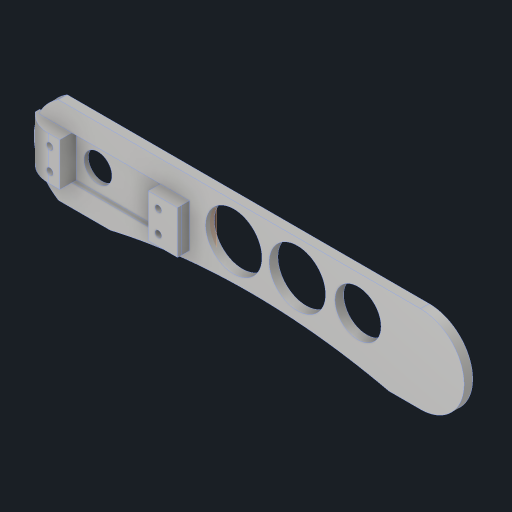
# Autodesk Inventor part: elbow
Saved by Autodesk Inventor 2023.4 (Build 274418000, 418)
## iProperties
Created: 2020-06-03
Part Number: elbow
Material: Aluminum 6061
Document SubType Name: Modeling
Designer: lenovo
Density: 2.7 g/cm^3
Appearance: Aluminum - Flat
Author: lenovo
Autodesk Inventor part; units mm, degrees
ref_plane "YZ Plane" through (0, 0, 0) normal (1, 0, 0) x (0, 1, 0)
ref_plane "XZ Plane" through (0, 0, 0) normal (0, 1, 0) x (-1, 0, 0)
ref_plane "XY Plane" through (0, 0, 0) normal (0, 0, 1) x (1, 0, 0)
sketch "Sketch1" plane through (0, 0, 0) normal (0, 0, 1) x (1, 0, 0)
  line L0 (-43.3376, 0) -> (106.6624, 0) construction
  line L1 (-43.3376, -20) -> (106.6624, -20)
  line L2 (106.6624, 20) -> (-43.3376, 20)
  arc A0 (-43.3376, 20) -> (-43.3376, -20) centre (-43.3376, 0) ccw
  arc A1 (106.6624, -20) -> (106.6624, 20) centre (106.6624, 0) ccw
  point P0 (0, 0)
  point P1 (31.6624, 0)
  dimension "d0" = 150
  dimension "d1" = 20
  constraints: 8 end point, 4 point on circle, 4 tangent, 2 centre point, 1 horizontal, 1 midpoint, 1 parallel
  measures "d0" distance of L0.end L0.start
  measures "d1" radius of A1
extrude "Extrusion1" add sketch "Sketch1" along normal blind 4
sketch "Sketch2" plane through (0, 0, 4) normal (0, 0, 1) x (1, 0, 0)
  arc A0 (-43.3376, 20) -> (-43.3376, -20) centre (-43.3376, 0) ccw projected
  arc A1 (106.6624, -20) -> (106.6624, 20) centre (106.6624, 0) ccw projected
  circle A2 centre (-43.3376, 0) radius 6.4
  circle A3 centre (106.6624, 0) radius 4
  point P0 (0, 0)
  dimension "d4" = 12.8
  dimension "d5" = 8
  constraints: 2 centre point, 2 coincident
  measures "d4" diameter of A2
  measures "d5" diameter of A3
extrude "Extrusion2" add sketch "Sketch2" against normal blind 11.9 contours A3
sketch "Sketch5" plane through (0, 0, 4) normal (0, 0, 1) x (1, 0, 0)
  line L0 (-43.3376, -20) -> (106.6624, -20) projected
  arc A0 (92.1536, -20) -> (-35.7554, -20) centre (28.1991, -294.1981) ccw
  point P0 (0, 0)
  constraints: 2 point on circle, 2 point on line, 1 centre point
extrude "Extrusion5" cut sketch "Sketch5" against normal through all
sketch "Sketch6" plane through (0, 0, 0) normal (0, 0, -1) x (-1, 0, 0)
  point P0 (0, 0)
sketch "Sketch7" plane through (106.6624, 0, -7.9) normal (0, 0, -1) x (-1, 0, 0)
  circle A0 centre (0, 0) radius 2.7
  point P0 (106.6624, 0)
  dimension "d18" = 5.4
  constraints: 1 centre point
  measures "d18" diameter of A0
extrude "Extrusion6" cut sketch "Sketch7" against normal blind 5
sketch "Sketch8" plane through (0, 0, 0) normal (0, 0, -1) x (-1, 0, 0)
  point P0 (0, 0)
extrude "Extrusion7" cut sketch "Sketch2" along normal mid plane 11.9 contours A2
sketch "Sketch9" plane through (106.6624, 0, -7.9) normal (0, 0, -1) x (-1, 0, 0)
  point P0 (106.6624, 0)
sketch "Sketch10" plane through (0, 0, 0) normal (0, 0, -1) x (-1, 0, 0)
  point P0 (0, 0)
sketch "Sketch11" plane through (0, 0, 4) normal (0, 0, 1) x (1, 0, 0)
  line L0 (-70.0866, 9.9) -> (0.6664, 9.9)
  line L1 (0.6664, 9.9) -> (0.6664, -9.9)
  line L2 (0.6664, -9.9) -> (-70.0866, -9.9)
  line L3 (-70.0866, -9.9) -> (-70.0866, 9.9)
  line L4 (-70.0866, 9.9) -> (0.6664, -9.9) construction
  line L5 (0.6664, 9.9) -> (-70.0866, -9.9) construction
  circle A0 centre (-43.3376, 0) radius 6.4 projected
  point P0 (0, 0)
  point P1 (-34.7101, 0)
  dimension "d23" = 70.753
  dimension "d24" = 19.8
  dimension "d25" = 26.749
  dimension "d26" = 9.9
  constraints: 12 end point, 2 midpoint, 2 parallel, 1 horizontal, 1 perpendicular
  measures "d23" distance of L1.end L2.end
  measures "d24" distance of L0.end L1.end
  measures "d25" distance from line of L3 A0.centre
  measures "d26" distance from line of L2 A0.centre
sketch "Sketch12" plane through (0, 0, 4) normal (0, 0, 1) x (1, 0, 0)
  circle A0 centre (-43.3376, 0) radius 6.4 projected
  point P0 (0, 0)
ref_plane "Work Plane1" through (0, 0, 2) normal (0, 0, 1) x (1, 0, 0)
sketch "Sketch13" plane through (0, 0, 2) normal (0, 0, 1) x (1, 0, 0)
  arc A0 (-43.3376, 20) -> (-60.7155, 9.9) centre (-43.3376, 0) ccw projected
  line L0 (-43.3376, 20) -> (-59.4218, 20)
  line L1 (-59.4166, -20.0032) -> (-43.3376, -20.0032)
  line L2 (-43.3376, -20.0032) -> (-43.3376, 20)
  circle A1 centre (-43.3376, 0) radius 4 projected
  arc A2 (-59.4218, 20) -> (-59.4166, -20.0032) centre (-47.3376, 0) ccw
  point P0 (0, 0)
  point P1 (-43.3376, -4)
  point P2 (-43.3376, 4)
  constraints: 6 end point, 2 point on circle, 1 centre point, 1 horizontal, 1 parallel, 2 other
extrude "Extrusion9" add sketch "Sketch13" along normal mid plane 4 contours L2 A1 L1 A2 L0
extrude "Extrusion10" cut sketch "Sketch11" against normal blind 2
sketch "Sketch14" plane through (0, 0, 2) normal (0, 0, 1) x (1, 0, 0)
  line L0 (-53.3376, 9.9) -> (-70.0866, 9.9)
  line L1 (-70.0866, 9.9) -> (-70.0866, -9.9)
  line L2 (-70.0866, -9.9) -> (-53.3376, -9.9)
  line L3 (-53.3376, -9.9) -> (-53.3376, 9.9)
  line L4 (-53.3376, 9.9) -> (-70.0866, -9.9) construction
  line L5 (-70.0866, 9.9) -> (-53.3376, -9.9) construction
  arc A0 (-43.3376, -6.4) -> (-43.3376, 6.4) centre (-43.3376, 0) ccw projected
  line L6 (-12.7376, 9.9) -> (0.6624, 9.9)
  line L7 (0.6624, 9.9) -> (0.6624, -9.9)
  line L8 (0.6624, -9.9) -> (-12.7376, -9.9)
  line L9 (-12.7376, -9.9) -> (-12.7376, 9.9)
  line L10 (-12.7376, 9.9) -> (0.6624, -9.9) construction
  line L11 (0.6624, 9.9) -> (-12.7376, -9.9) construction
  point P0 (0, 0)
  point P1 (-61.7121, 0)
  point P2 (-61.7121, -9.9)
  point P3 (-6.0376, 0)
  dimension "d33" = 19.8
  dimension "d34" = 16.749
  dimension "d35" = 10
  dimension "d36" = 13.4
  dimension "d37" = 19.8
  dimension "d38" = 30.6
  constraints: 24 end point, 5 midpoint, 4 parallel, 2 horizontal, 2 perpendicular
  measures "d33" distance from line of point (-61.712, -9.9) L0
  measures "d34" distance between parallel lines of L1 L3
  measures "d35" distance from line of A0.centre L3
  measures "d36" distance of L7.end L8.end
  measures "d37" distance of L6.end L7.end
  measures "d38" distance from line of A0.centre L9
extrude "Extrusion11" add sketch "Sketch14" along normal blind 7.5
fillet "Fillet3" radius 14.75 1 edges at (-70.0866, 0, 9.5)
sketch "Sketch15" plane through (0, 0, 2) normal (0, 0, 1) x (1, 0, 0)
  line L0 (0.6664, -9.9) -> (0.6624, -9.9) projected
  line L1 (0.6664, 9.9) -> (0.6664, -9.9) projected
  line L2 (0.6624, -9.9) -> (0.6664, -9.9)
  line L3 (0.6664, -9.9) -> (0.6664, 9.9)
  line L4 (0.6664, 9.9) -> (0.6624, 9.9)
  line L5 (0.6624, 9.9) -> (0.6624, -9.9)
  point P0 (0, 0)
  constraints: 8 end point, 2 parallel, 1 horizontal, 1 perpendicular
extrude "Extrusion12" add sketch "Sketch15" along normal blind 5.5
sketch "Sketch16" plane through (0, 0, 9.5) normal (0, 0, 1) x (1, 0, 0)
  circle A0 centre (-57.9276, -5) radius 1.475
  circle A1 centre (-57.9276, 5) radius 1.475
  line L0 (-58.5975, -9.9) -> (-58.5975, 9.9) projected
  line L1 (-58.5975, -9.9) -> (-53.3376, -9.9) projected
  line L2 (-53.3376, 9.9) -> (-58.5975, 9.9) projected
  circle A2 centre (-8.1476, -5) radius 1.475
  circle A3 centre (-8.1476, 5) radius 1.475
  line L3 (-12.7376, 9.9) -> (-12.7376, -9.9) projected
  line L4 (-12.7376, -9.9) -> (0.6664, -9.9) projected
  line L5 (0.6664, 9.9) -> (-12.7376, 9.9) projected
  arc A4 (-43.3376, -6.4) -> (-43.3376, 6.4) centre (-43.3376, 0) ccw projected
  point P0 (0, 0)
  dimension "d44" = 2.95
  dimension "d45" = 2.95
  dimension "d47" = 4.9
  dimension "d49" = 4.9
  dimension "d50" = 2.95
  dimension "d51" = 2.95
  dimension "d52" = 4.59
  dimension "d53" = 4.59
  dimension "d54" = 4.9
  dimension "d55" = 4.9
  dimension "d60" = 14.59
  dimension "d61" = 14.59
  constraints: 4 centre point
  measures "d44" diameter of A0
  measures "d45" diameter of A1
  measures "d47" distance from line of L1 A0.centre
  measures "d49" distance from line of L2 A1.centre
  measures "d50" diameter of A2
  measures "d51" diameter of A3
  measures "d52" distance from line of L3 A2.centre
  measures "d53" distance from line of L3 A3.centre
  measures "d54" distance from line of L4 A2.centre
  measures "d55" distance from line of L5 A3.centre
  measures "d60" horizontal distance of A4.centre A0.centre
  measures "d61" horizontal distance of A4.centre A1.centre
extrude "Extrusion13" cut sketch "Sketch16" against normal blind 10
sketch "Sketch17" plane through (0, 0, 2) normal (0, 0, 1) x (1, 0, 0)
  point P0 (0, 0)
sketch "Sketch18" plane through (0, 0, 2) normal (0, 0, 1) x (1, 0, 0)
  point P0 (0, 0)
extrude "Extrusion14" cut sketch "Sketch12" against normal blind 11.9
sketch "Sketch19" plane through (0, 0, 4) normal (0, 0, 1) x (1, 0, 0)
  circle A0 centre (20.9836, 3.8774) radius 12.933
  circle A1 centre (50.1781, 3.8774) radius 12.933
  circle A2 centre (77.9924, 3.8774) radius 10.5714
  point P0 (0, 0)
  constraints: 3 centre point
extrude "Extrusion15" cut sketch "Sketch19" against normal blind 10
sketch "Sketch20" plane through (0, 0, 2) normal (0, 0, 1) x (1, 0, 0)
  point P0 (0, 0)
body "Solid1"
